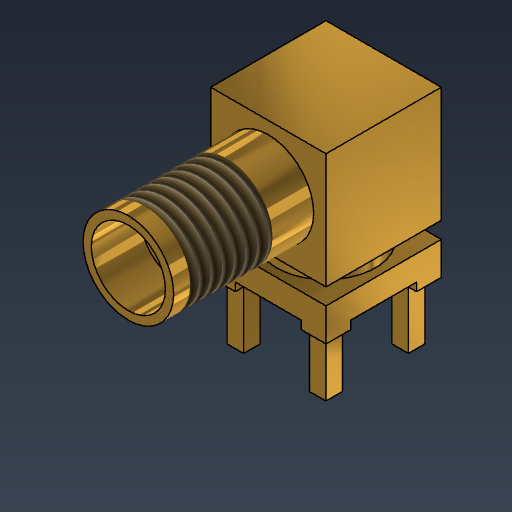
# Autodesk Inventor part: SMA-F-RA
Saved by Autodesk Inventor 2023.1 (Build 271208000, 208)
## iProperties
Created: 2017-11-11
Part Number: SMA-F-RA
Material: Messing, weicher Gelbton
Document SubType Name: Modeling
Designer: rYan
Density: 8.47 g/cm^3
Appearance: Messing - satiniert
Mass: 5.24079 g
Surface Area: 6.72117 cm^2
Volume: 0.618748 cm^3
Author: rYan
Autodesk Inventor part; units mm, degrees
ref_plane "YZ Plane" through (0, 0, 0) normal (1, 0, 0) x (0, 1, 0)
ref_plane "XZ Plane" through (0, 0, 0) normal (0, 1, 0) x (-1, 0, 0)
ref_plane "XY Plane" through (0, 0, 0) normal (0, 0, 1) x (1, 0, 0)
sketch "Skizze1" plane through (0, 0, 0) normal (0, 0, 1) x (1, 0, 0)
  line L0 (-3.5, -3.5) -> (3.5, -3.5)
  line L1 (3.5, -3.5) -> (3.5, 3.5)
  line L2 (3.5, 3.5) -> (-3.5, 3.5)
  line L3 (-3.5, 3.5) -> (-3.5, -3.5)
  line L4 (-3.5, -3.5) -> (3.5, 3.5) construction
  line L5 (3.5, -3.5) -> (-3.5, 3.5) construction
  point P0 (0, 0)
  dimension "d0" = 7
  dimension "d1" = 7
  constraints: 12 end point, 2 midpoint, 2 parallel, 1 horizontal, 1 perpendicular
  measures "d0" distance of L2.end L1.end
  measures "d1" distance of L1.end L0.end
extrude "Extrusion1" add sketch "Skizze1" along normal blind 7
sketch "Skizze2" plane through (0, 0, 0) normal (0, 0, -1) x (-1, 0, 0)
  circle A0 centre (0, 0) radius 3
  dimension "d4" = 6
  constraints: 1 centre point, 1 coincident
  measures "d4" diameter of A0
extrude "Extrusion2" add sketch "Skizze2" along normal blind 1
sketch "Skizze3" plane through (0, 0, -1) normal (0, 0, -1) x (-1, 0, 0)
  line L0 (3.5, 3.5) -> (-3.5, 3.5)
  line L1 (-3.5, 3.5) -> (-3.5, -3.5)
  line L2 (-3.5, -3.5) -> (3.5, -3.5)
  line L3 (3.5, -3.5) -> (3.5, 3.5)
  line L4 (3.5, 3.5) -> (-3.5, -3.5) construction
  line L5 (-3.5, 3.5) -> (3.5, -3.5) construction
  point P0 (0, 0)
  dimension "d7" = 7
  dimension "d8" = 7
  constraints: 12 end point, 2 midpoint, 2 parallel, 1 horizontal, 1 perpendicular
  measures "d7" distance of L2.end L1.end
  measures "d8" distance of L1.end L0.end
extrude "Extrusion3" add sketch "Skizze3" along normal blind 1.5
sketch "Skizze4" plane through (0, 0, -2.5) normal (0, 0, -1) x (-1, 0, 0)
  line L0 (3.5, 3.5) -> (-3.5, 3.5) projected
  line L1 (-3.5, 3.5) -> (-3.5, -3.5) projected
  line L2 (-3.5, -3.5) -> (3.5, -3.5) projected
  line L3 (3.5, -3.5) -> (3.5, 3.5) projected
  line L4 (-3.5, 3.5) -> (3.5, 3.5) projected
  line L5 (3.5, 3.5) -> (2, 3.5)
  line L6 (2, 3.5) -> (2, 2)
  line L7 (2, 2) -> (3.5, 2)
  line L8 (3.5, 2) -> (3.5, 3.5)
  line L9 (3.5, -3.5) -> (-3.5, -3.5) projected
  line L10 (3.5, -3.5) -> (2, -3.5)
  line L11 (2, -3.5) -> (2, -2)
  line L12 (2, -2) -> (3.5, -2)
  line L13 (3.5, -2) -> (3.5, -3.5)
  line L14 (-3.5, 3.5) -> (-2, 3.5)
  line L15 (-2, 3.5) -> (-2, 2)
  line L16 (-2, 2) -> (-3.5, 2)
  line L17 (-3.5, 2) -> (-3.5, 3.5)
  line L18 (-3.5, -3.5) -> (-3.5, 3.5) projected
  line L19 (-3.5, -3.5) -> (-2, -3.5)
  line L20 (-2, -3.5) -> (-2, -2)
  line L21 (-2, -2) -> (-3.5, -2)
  line L22 (-3.5, -2) -> (-3.5, -3.5)
  point P0 (0, 0)
  dimension "d11" = 1.5
  dimension "d12" = 1.5
  dimension "d13" = 1.5
  dimension "d14" = 1.5
  dimension "d15" = 1.5
  dimension "d16" = 1.5
  dimension "d17" = 1.5
  dimension "d18" = 1.5
  constraints: 32 end point, 8 parallel, 4 horizontal, 4 perpendicular
  measures "d11" distance of L7.end L6.end
  measures "d12" distance of L6.end L5.end
  measures "d13" distance of L11.end L12.end
  measures "d14" distance of L10.end L11.end
  measures "d15" distance of L15.end L16.end
  measures "d16" distance of L14.end L15.end
  measures "d17" distance of L21.end L20.end
  measures "d18" distance of L20.end L19.end
extrude "Extrusion4" add sketch "Skizze4" along normal blind 0.5 contours L3 L7 L6 L0 | L15 L16 L1 L0 | L3 L2 L11 L12 | L21 L20 L2 L1
sketch "Skizze5" plane through (0, 0, -3) normal (0, 0, -1) x (-1, 0, 0)
  line L0 (3.5, -3.5) -> (3.5, -2) projected
  line L1 (3.5, -2) -> (2, -2) projected
  line L2 (2, -2) -> (2, -3.5) projected
  line L3 (2, -3.5) -> (3.5, -3.5) projected
  line L4 (-3.5, -3.5) -> (-2, -3.5) projected
  line L5 (-2, -3.5) -> (-2, -2) projected
  line L6 (-2, -2) -> (-3.5, -2) projected
  line L7 (-3.5, -2) -> (-3.5, -3.5) projected
  line L8 (-3.5, 3.5) -> (-3.5, 2) projected
  line L9 (-3.5, 2) -> (-2, 2) projected
  line L10 (-2, 2) -> (-2, 3.5) projected
  line L11 (-2, 3.5) -> (-3.5, 3.5) projected
  line L12 (3.5, 3.5) -> (2, 3.5) projected
  line L13 (2, 3.5) -> (2, 2) projected
  line L14 (2, 2) -> (3.5, 2) projected
  line L15 (3.5, 2) -> (3.5, 3.5) projected
  line L16 (2, -2) -> (3, -2)
  line L17 (3, -2) -> (3, -3)
  line L18 (3, -3) -> (2, -3)
  line L19 (2, -3) -> (2, -2)
  line L20 (-2, -2) -> (-3, -2)
  line L21 (-3, -2) -> (-3, -3)
  line L22 (-3, -3) -> (-2, -3)
  line L23 (-2, -3) -> (-2, -2)
  line L24 (-2, 2) -> (-3, 2)
  line L25 (-3, 2) -> (-3, 3)
  line L26 (-3, 3) -> (-2, 3)
  line L27 (-2, 3) -> (-2, 2)
  line L28 (2, 2) -> (3, 2)
  line L29 (3, 2) -> (3, 3)
  line L30 (3, 3) -> (2, 3)
  line L31 (2, 3) -> (2, 2)
  point P0 (0, 0)
  dimension "d21" = 1
  dimension "d22" = 1
  dimension "d23" = 1
  dimension "d24" = 1
  dimension "d25" = 1
  dimension "d26" = 1
  dimension "d27" = 1
  dimension "d28" = 1
  constraints: 32 end point, 8 parallel, 4 horizontal, 4 perpendicular
  measures "d21" distance of L17.end L18.end
  measures "d22" distance of L16.end L17.end
  measures "d23" distance of L22.end L21.end
  measures "d24" distance of L21.end L20.end
  measures "d25" distance of L25.end L26.end
  measures "d26" distance of L24.end L25.end
  measures "d27" distance of L30.end L29.end
  measures "d28" distance of L29.end L28.end
extrude "Extrusion5" add sketch "Skizze5" along normal blind 3.5 contours L17 L18 L2 L1 | L22 L21 L6 L5 | L25 L26 L10 L9 | L30 L29 L14 L13
sketch "Skizze6" plane through (0, 0, -2.5) normal (0, 0, -1) x (-1, 0, 0)
  circle A0 centre (0, 0) radius 0.5
  dimension "d31" = 1
  constraints: 1 centre point, 1 coincident
  measures "d31" diameter of A0
extrude "Extrusion6" add sketch "Skizze6" along normal blind 3.5
sketch "Skizze7" plane through (-3.5, -3.5, 0) normal (0, -1, 0) x (1, 0, 0)
  line L0 (0, 0) -> (7, 0) projected
  line L1 (7, 0) -> (7, 7) projected
  line L2 (0, 7) -> (7, 7) projected
  line L3 (0, 0) -> (0, 7) projected
  line L4 (0, 0) -> (0, 7) construction
  line L5 (0, 3.5) -> (7, 3.5) construction
  line L6 (3.5, 7) -> (3.5, 0) construction
  circle A0 centre (3.5, 3.5) radius 2.75
  dimension "d34" = 5.5
  constraints: 4 end point, 4 midpoint, 1 centre point, 1 vertical
  measures "d34" diameter of A0
extrude "Extrusion7" add sketch "Skizze7" along normal blind 8.5 contours A0
thread "Gewinde1" size "1/4-36 UNS" class "2A" standard "ANSI Unified Screw Threads" length 5 offset 1
sketch "Skizze8" plane through (0, -12, 3.5) normal (0, -1, 0) x (1, 0, 0)
  circle A0 centre (0, 0) radius 2.75 projected
  circle A1 centre (0, 0) radius 2.25
  point P0 (0, -3.5)
  dimension "d39" = 4.5
  constraints: 1 centre point, 1 coincident
  measures "d39" diameter of A1
extrude "Extrusion8" cut sketch "Skizze8" against normal blind 3 contours A1
sketch "Skizze9" plane through (0, -9, 3.5) normal (0, -1, 0) x (1, 0, 0)
  circle A0 centre (0, 0) radius 2.25 projected
  circle A1 centre (0, 0) radius 0.4
  point P0 (0, -3.5)
  dimension "d42" = 0.8
  constraints: 1 centre point, 1 coincident
  measures "d42" diameter of A1
extrude "Extrusion9" cut sketch "Skizze9" against normal blind 3 contours A1
